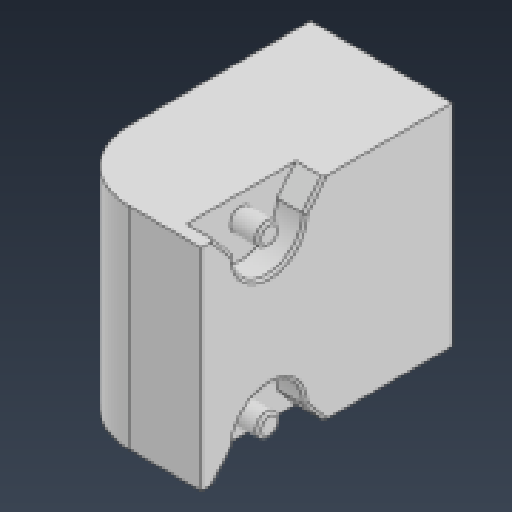
# Autodesk Inventor part: front-lunad-holder
Saved by Autodesk Inventor 2023 (Build 270158000, 158)
## iProperties
Created: 2025-04-06
Part Number: front-lunad-holder
Material: Generic
Document SubType Name: Modeling
Designer: szymo
Density: 1 g/cm^3
Appearance: Default
Author: szymo
Autodesk Inventor part; units mm, degrees
ref_plane "YZ Plane" through (0, 0, 0) normal (1, 0, 0) x (0, 1, 0)
ref_plane "XZ Plane" through (0, 0, 0) normal (0, 1, 0) x (-1, 0, 0)
ref_plane "XY Plane" through (0, 0, 0) normal (0, 0, 1) x (1, 0, 0)
ref_plane "Work Plane1" through (0, 0, 0) normal (0, 0, 1) x (1, 0, 0)
sketch "Sketch1" plane through (0, 0, 0) normal (0, 0, 1) x (1, 0, 0)
  line L0 (-33.9, 7.85) -> (-44.9, 7.85) projected
  line L1 (-35.9, 5.925) -> (-35.9, 7.85) projected
  line L2 (-35.9, 5.925) -> (-35.9, 3.675) projected
  line L3 (-35.9, -7.85) -> (-35.9, -5.925) projected
  line L4 (-35.9, -3.675) -> (-35.9, -5.925) projected
  line L5 (-44.9, -7.85) -> (-33.9, -7.85) projected
  line L6 (-33.9, 7.55) -> (-44.0855, 7.55)
  line L7 (-44.0855, -7.55) -> (-33.9, -7.55)
  line L8 (-39.5, 49.5) -> (-39.5, 38.5) projected
  line L9 (-39.5, 7.55) -> (-39.5, -7.55)
  line L10 (-33.9, 5.925) -> (-33.9, 3.675) projected
  line L11 (-33.9, 5.925) -> (-33.9, 7.85) projected
  line L12 (-35.9, 3.675) -> (-33.9, 3.675)
  line L13 (-33.9, -7.85) -> (-33.9, -5.925) projected
  line L14 (-33.9, -3.675) -> (-33.9, -5.925) projected
  line L15 (-35.9, -3.675) -> (-33.9, -3.675)
  line L16 (-33.9, 3.675) -> (-33.9, -3.675)
  line L17 (-35.9, -3.675) -> (-35.9, 3.675)
  line L18 (-44.0855, -38.5) -> (-44.0855, 38.5) projected
  point P0 (0, 0)
  point P1 (-35.9, 7.55)
  point P2 (-35.9, -7.55)
  dimension "d0" = 0.3
  dimension "d1" = 0.3
  constraints: 14 end point, 6 point on line, 3 parallel, 2 horizontal, 1 collinear
  measures "d0" distance between parallel lines of L0 L6
  measures "d1" distance between parallel lines of L5 L7
extrude "Extrusion1" add sketch "Sketch1" along normal blind 18 contours L11 L10 L12 L2 L1 L6 | L1 L2 L17 L4 L3 L7 L9 L6 | L6 L9 L7 L18 | L16 L15 L17 L12 | L14 L13 L7 L3 L4 L15
sketch "Sketch2" plane through (-33.9, -7.55, 0) normal (1, 0, 0) x (0, 0, -1)
  line L0 (-2, -8.375) -> (-1, -8.375) projected
  line L1 (-1, -5.125) -> (-1, -8.375) projected
  arc A0 (-1, -5.125) -> (-1.5, -4.625) centre (-1.5, -5.125) ccw projected
  line L2 (-1.5, -4.625) -> (-2.6534, -4.625) projected
  arc A1 (-3.153, -4.1444) -> (-2.6534, -4.625) centre (-2.6534, -4.125) ccw projected
  arc A2 (-3.153, -4.1444) -> (-7.15, -0.3) centre (-7.15, -4.3) ccw projected
  line L3 (-9.2847, -0.3) -> (-7.15, -0.3) projected
  line L4 (-10.9, 1.625) -> (-9.2847, -0.3) projected
  arc A3 (-10.9, 1.625) -> (-15.4, 1.625) centre (-13.15, 1.625) ccw projected
  line L5 (-17.0153, -0.3) -> (-15.4, 1.625) projected
  line L6 (-17.15, -0.3) -> (-17.0153, -0.3) projected
  arc A4 (-17.15, -0.3) -> (-22.15, -5.3) centre (-17.15, -5.3) ccw projected
  line L7 (-22.15, -21.95) -> (-22.15, -5.3) projected
  arc A5 (-22.15, -21.95) -> (-17.15, -26.95) centre (-17.15, -21.95) ccw projected
  line L8 (-17.0153, -26.95) -> (-17.15, -26.95) projected
  line L9 (-15.4, -28.875) -> (-17.0153, -26.95) projected
  arc A6 (-15.4, -28.875) -> (-10.9, -28.875) centre (-13.15, -28.875) ccw projected
  line L10 (-9.2847, -26.95) -> (-10.9, -28.875) projected
  line L11 (-7.15, -26.95) -> (-9.2847, -26.95) projected
  arc A7 (-7.15, -26.95) -> (-3.153, -23.1056) centre (-7.15, -22.95) ccw projected
  arc A8 (-2.6534, -22.625) -> (-3.153, -23.1056) centre (-2.6534, -23.125) ccw projected
  line L12 (-1.5, -22.625) -> (-2.6534, -22.625) projected
  arc A9 (-1.5, -22.625) -> (-1, -22.125) centre (-1.5, -22.125) ccw projected
  line L13 (-1, -18.875) -> (-1, -22.125) projected
  line L14 (-2, -18.875) -> (-1, -18.875) projected
  line L15 (-2, -8.375) -> (-2, -18.875) projected
  circle A10 centre (-13.15, 1.625) radius 1.1 projected
  circle A11 centre (-13.15, -28.875) radius 1.1 projected
  line L16 (-2, 33.975) -> (-1, 33.975) projected
  line L17 (-1, 37.225) -> (-1, 33.975) projected
  arc A12 (-1, 37.225) -> (-1.5, 37.725) centre (-1.5, 37.225) ccw projected
  line L18 (-1.5, 37.725) -> (-2.6534, 37.725) projected
  arc A13 (-3.153, 38.2056) -> (-2.6534, 37.725) centre (-2.6534, 38.225) ccw projected
  arc A14 (-3.153, 38.2056) -> (-7.15, 42.05) centre (-7.15, 38.05) ccw projected
  line L19 (-9.2847, 42.05) -> (-7.15, 42.05) projected
  line L20 (-10.9, 43.975) -> (-9.2847, 42.05) projected
  arc A15 (-10.9, 43.975) -> (-15.4, 43.975) centre (-13.15, 43.975) ccw projected
  line L21 (-17.0153, 42.05) -> (-15.4, 43.975) projected
  line L22 (-17.15, 42.05) -> (-17.0153, 42.05) projected
  arc A16 (-17.15, 42.05) -> (-22.15, 37.05) centre (-17.15, 37.05) ccw projected
  line L23 (-22.15, 20.4) -> (-22.15, 37.05) projected
  arc A17 (-22.15, 20.4) -> (-17.15, 15.4) centre (-17.15, 20.4) ccw projected
  line L24 (-17.0153, 15.4) -> (-17.15, 15.4) projected
  line L25 (-15.4, 13.475) -> (-17.0153, 15.4) projected
  arc A18 (-15.4, 13.475) -> (-10.9, 13.475) centre (-13.15, 13.475) ccw projected
  line L26 (-9.2847, 15.4) -> (-10.9, 13.475) projected
  line L27 (-7.15, 15.4) -> (-9.2847, 15.4) projected
  arc A19 (-7.15, 15.4) -> (-3.153, 19.2444) centre (-7.15, 19.4) ccw projected
  arc A20 (-2.6534, 19.725) -> (-3.153, 19.2444) centre (-2.6534, 19.225) ccw projected
  line L28 (-1.5, 19.725) -> (-2.6534, 19.725) projected
  arc A21 (-1.5, 19.725) -> (-1, 20.225) centre (-1.5, 20.225) ccw projected
  line L29 (-1, 23.475) -> (-1, 20.225) projected
  line L30 (-2, 23.475) -> (-1, 23.475) projected
  line L31 (-2, 33.975) -> (-2, 23.475) projected
  circle A22 centre (-13.15, 43.975) radius 1.1 projected
  circle A23 centre (-13.15, 13.475) radius 1.1 projected
  line L32 (0, 0) -> (0, 15.1) projected
  line L33 (0, 15.1) -> (-18, 15.1) projected
  line L34 (-18, 0) -> (-18, 15.1) projected
  line L35 (0, 0) -> (-18, 0) projected
  circle A24 centre (-13.15, 1.625) radius 2.55
  circle A25 centre (-13.15, 13.475) radius 2.55
  line L36 (0, 0) -> (-18, 0) projected
  line L37 (-15.7, 13.475) -> (-17.0635, 15.1)
  line L38 (-10.6, 13.475) -> (-8.9847, 15.4)
  line L39 (-10.6, 1.625) -> (-8.9847, -0.3)
  line L40 (-10.6, 1.625) -> (-10.9, 1.625)
  line L41 (-17.0635, 0) -> (-15.7, 1.625)
  line L42 (-15.7, 1.625) -> (-15.4, 1.625)
  line L43 (-15.4, 13.475) -> (-15.7, 13.475)
  line L44 (-10.9, 13.475) -> (-10.6, 13.475)
  circle A26 centre (-13.15, 1.625) radius 0.8
  circle A27 centre (-13.15, 13.475) radius 0.8
  point P0 (0, 7.55)
  point P1 (-16.7635, 0)
  point P2 (-9.5365, 0)
  point P3 (-9.2365, 15.1)
  point P4 (-9.2365, 0)
  dimension "d34" = 0.3
  dimension "d35" = 0.3
  dimension "d36" = 0.3
  dimension "d37" = 0.3
  constraints: 16 end point, 8 point on line, 4 centre point, 4 horizontal, 4 parallel, 4 point on circle, 2 coincident
  measures "d34" radial gap between concentric circles of A24 A3
  measures "d35" radial gap between concentric circles of A25 A18
  measures "d36" radial gap between concentric circles of A26 A10
  measures "d37" radial gap between concentric circles of A23 A27
extrude "Extrusion2" cut sketch "Sketch2" against normal blind 2 contours L35 L4 A24 L39 | L35 A24 L4 | L40 A3 L42 A24 | A24 L4 L40 | A24 L35 L5 A3 L4 | L42 L5 A24 | A24 L5 L35 L41 | L35 L5 A24 | L38 A25 L26 L33 | L26 A25 L33 | L44 L26 A25 | A25 L43 A18 L44 | L26 A18 L25 A25 L33 | L37 L33 L25 A25 | A25 L25 L43 | A25 L25 L33 | A10 | A23
fillet "Fillet1" radius 0.2 8 edges at (-33.9, -3.375, 13.15) (-33.9, -6.7375, 16.3818) (-33.9, -6.7375, 9.9182) (-33.9, 6.7375, 9.9182) (-33.9, 3.375, 13.15) (-33.9, 6.7375, 16.3818) (-33.9, -5.925, 13.95) (-33.9, 5.925, 13.95)
fillet "Fillet2" radius 5 1 edges at (-44.0855, 0, 18)
sketch "Sketch4" plane through (0, 0, 0) normal (0, 0, -1) x (-1, 0, 0)
  line L0 (44.0855, -7.55) -> (33.9, -7.55) construction
  line L1 (44.0855, 7.55) -> (44.0855, -7.55) construction
  line L2 (33.9, 7.55) -> (44.0855, 7.55) construction
  line L3 (38.0855, -7.55) -> (38.0855, 7.55) construction
  line L4 (38.0855, 0) -> (44.0855, 0) construction
  line L5 (44.0855, 0) -> (38.0855, -7.55) construction
  line L6 (44.0855, -7.55) -> (38.0855, 0) construction
  line L7 (38.0855, 0) -> (44.0855, 7.55) construction
  line L8 (38.0855, 7.55) -> (44.0855, 0) construction
  line L9 (33.9, -7.55) -> (33.9, 7.55) projected
  point P0 (0, 0)
  point P1 (41.0855, 3.775)
  point P2 (41.0855, -3.775)
  dimension "d26" = 6
  constraints: 12 end point, 4 midpoint, 2 parallel, 1 perpendicular, 1 point on line
  measures "d26" distance between parallel lines of L1 L3
hole "Hole2" at (-41.0855, -3.775, 0) at (-41.0855, 3.775, 0) direction (0, 0, 1) diameter 4 depth 5.5 counterbore diameter 5 counterbore depth 0.5
sketch "Sketch5" plane through (-41.0855, -3.775, 5.5) normal (0, 0, -1) x (-1, 0, 0)
  circle A0 centre (0, 0) radius 2 projected
  circle A1 centre (0, 7.55) radius 2 projected
  circle A2 centre (0, 0) radius 2 projected
  point P0 (-41.0855, 3.775)
  constraints: 2 coincident
hole "Hole3" at (-41.0855, 3.775, 5.5) at (-41.0855, -3.775, 5.5) direction (0, 0, 1) diameter 3.1 depth 9 countersink diameter 4 countersink angle 90
body "Solid1"
